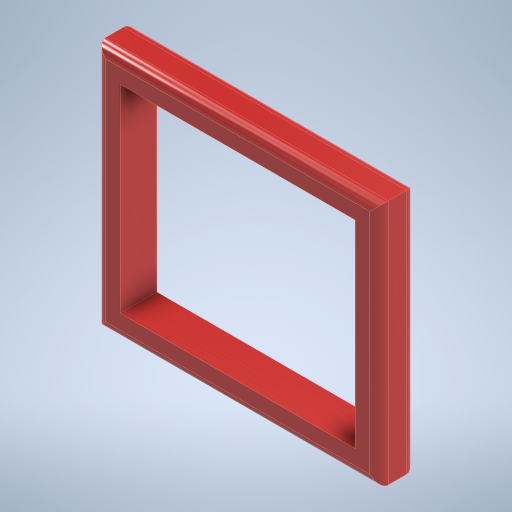
# Autodesk Inventor part: Red Bumper
Saved by Autodesk Inventor 2023 (Build 270158030, 158C)
## iProperties
Created: 2022-07-18
Part Number: Red Bumper
Material: Generic
Document SubType Name: Modeling
Designer: bk0872852
Density: 1 g/cm^3
Appearance: Orange-Red
Author: bk0872852
Autodesk Inventor part; units mm, degrees
ref_plane "YZ Plane" through (0, 0, 0) normal (1, 0, 0) x (0, 1, 0)
ref_plane "XZ Plane" through (0, 0, 0) normal (0, 1, 0) x (-1, 0, 0)
ref_plane "XY Plane" through (0, 0, 0) normal (0, 0, 1) x (1, 0, 0)
sketch "Sketch1" plane through (0, 0, 0) normal (0, 0, 1) x (1, 0, 0)
  line L0 (-396.3923, 183.6197) -> (416.4077, 183.6197)
  line L1 (416.4077, 183.6197) -> (416.4077, -502.1803)
  line L2 (416.4077, -502.1803) -> (-396.3923, -502.1803)
  line L3 (-396.3923, -502.1803) -> (-396.3923, 183.6197)
  line L4 (498.9577, 266.1697) -> (-478.9423, 266.1697)
  line L5 (-478.9423, 266.1697) -> (-478.9423, -584.7303)
  line L6 (-478.9423, -584.7303) -> (498.9577, -584.7303)
  line L7 (498.9577, -584.7303) -> (498.9577, 266.1697)
  point P0 (0, 0)
  dimension "d0" = 812.8
  dimension "d1" = 685.8
  dimension "d2" = 82.55
  constraints: 16 end point, 4 parallel, 2 perpendicular, 1 horizontal, 3 other
  measures "d0" distance of L0.start L0.end
  measures "d1" distance of L2.end L0.start
  measures "d2" distance between parallel lines of L0 L4
extrude "Extrusion1" add sketch "Sketch1" along normal blind 127
fillet "Fillet1" radius 31.75 8 edges at (10.0077, 266.1697, 127) (-478.9423, -159.2803, 127) (10.0077, -584.7303, 127) (498.9577, -159.2803, 127) (498.9577, -159.2803, 0) (10.0077, 266.1697, 0) (10.0077, -584.7303, 0) (-478.9423, -159.2803, 0)
body "Solid1"
